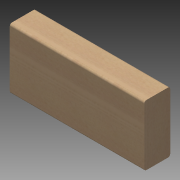
# Autodesk Inventor part: 2x4x7.75
Saved by Autodesk Inventor 2014 (Build 180170000, 170)
## iProperties
Created: 2013-10-13
Part Number: 2x4x7.75
Material: Ash
Document SubType Name: Modeling
Designer: david
Density: 0.641 g/cm^3
Appearance: Ash Door
Author: david
Autodesk Inventor part; units mm, degrees
ref_plane "YZ Plane" through (0, 0, 0) normal (1, 0, 0) x (0, 1, 0)
ref_plane "XZ Plane" through (0, 0, 0) normal (0, 1, 0) x (-1, 0, 0)
ref_plane "XY Plane" through (0, 0, 0) normal (0, 0, 1) x (1, 0, 0)
sketch "Sketch1" plane through (0, 0, 0) normal (1, 0, 0) x (0, 1, 0)
  line L0 (-3.7488, 0) -> (85.1512, 0)
  line L1 (85.1512, 0) -> (85.1512, 38.1)
  line L2 (85.1512, 38.1) -> (-3.7488, 38.1)
  line L3 (-3.7488, 38.1) -> (-3.7488, 0)
  point P0 (0, 0)
  dimension "d0" = 88.9
  dimension "d1" = 38.1
  constraints: 8 end point, 2 parallel, 1 horizontal, 1 perpendicular
  measures "d0" distance of L0.start L0.end
  measures "d1" distance of L2.end L0.start
extrude "Extrusion1" add sketch "Sketch1" along normal blind 196.85
fillet "Fillet1" radius 3.175 4 edges at (98.425, 85.1512, 38.1) (98.425, 85.1512, 0) (98.425, -3.7488, 0) (98.425, -3.7488, 38.1)
body "Solid1"
